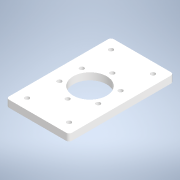
# Autodesk Inventor part: MotorBracket
Saved by Autodesk Inventor 2021 (Build 250183000, 183)
## iProperties
Created: 2021-05-22
Part Number: MotorBracket
Material: PC/ABS Plastic
Document SubType Name: Modeling
Designer: sami8
Density: 0.357273 g/cm^3
Appearance: Smooth - White
Author: sami8
Autodesk Inventor part; units mm, degrees
ref_plane "YZ Plane" through (0, 0, 0) normal (1, 0, 0) x (0, 1, 0)
ref_plane "XZ Plane" through (0, 0, 0) normal (0, 1, 0) x (-1, 0, 0)
ref_plane "XY Plane" through (0, 0, 0) normal (0, 0, 1) x (1, 0, 0)
sketch "Sketch1" plane through (0, 0, 0) normal (0, 1, 0) x (-1, 0, 0)
  circle A0 centre (0, 0) radius 12
  line L0 (22.5, 37.5) -> (-22.5, 37.5)
  line L1 (-22.5, 37.5) -> (-22.5, -37.5)
  line L2 (-22.5, -37.5) -> (22.5, -37.5)
  line L3 (22.5, -37.5) -> (22.5, 37.5)
  line L4 (22.5, 37.5) -> (-22.5, -37.5) construction
  line L5 (-22.5, 37.5) -> (22.5, -37.5) construction
  circle A1 centre (0, 0) radius 16 construction
  line L6 (0, 0) -> (0, -16) construction
  circle A2 centre (0, -16) radius 1.55
  circle A3 centre (13.8564, -8) radius 1.55
  circle A4 centre (13.8564, 8) radius 1.55
  circle A5 centre (0, 16) radius 1.55
  circle A6 centre (-13.8564, 8) radius 1.55
  circle A7 centre (-13.8564, -8) radius 1.55
  line L7 (15, -30) -> (-15, -30) construction
  line L8 (-15, -30) -> (-15, 30) construction
  line L9 (-15, 30) -> (15, 30) construction
  line L10 (15, 30) -> (15, -30) construction
  line L11 (15, -30) -> (-15, 30) construction
  line L12 (-15, -30) -> (15, 30) construction
  circle A8 centre (15, -30) radius 1.55
  circle A9 centre (-15, -30) radius 1.55
  circle A10 centre (15, 30) radius 1.55
  circle A11 centre (-15, 30) radius 1.55
  dimension "d3" = 32
  dimension "d0" = 24
  dimension "d1" = 45
  dimension "d2" = 75
  dimension "d4" = 3.1
  dimension "d7" = 360
  dimension "d12" = 30
  dimension "d13" = 60
  dimension "d14" = 3.1
  dimension "d15" = 3.1
  dimension "d16" = 3.1
  dimension "d17" = 3.1
  constraints: 26 end point, 11 centre point, 7 coincident, 4 midpoint, 4 parallel, 2 horizontal, 2 perpendicular, 1 vertical, 1 vertical alignment, 15 other
  measures "d0" diameter of A0
  measures "d1" distance of L2.end L1.end
  measures "d2" distance of L1.end L0.end
  measures "d4" diameter of A2
  measures "d12" distance of L8.end L9.end
  measures "d13" distance of L7.end L8.end
  measures "d14" diameter of A8
  measures "d15" diameter of A9
  measures "d16" diameter of A10
  measures "d17" diameter of A11
extrude "Extrusion1" add sketch "Sketch1" along normal blind 5
fillet "Fillet1" radius 2 4 edges at (22.5, 2.5, 37.5) (-22.5, 2.5, 37.5) (-22.5, 2.5, -37.5) (22.5, 2.5, -37.5)
body "Solid1"
